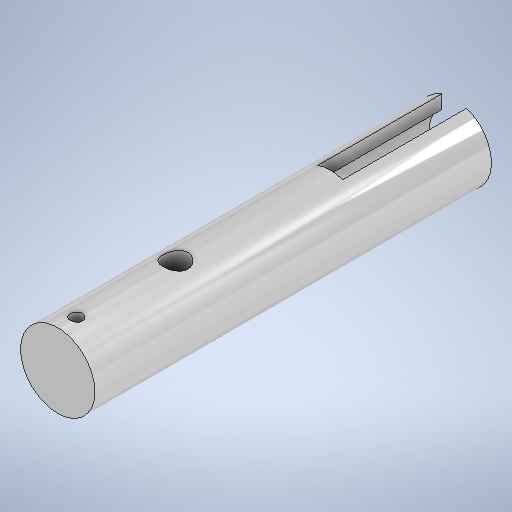
# Autodesk Inventor part: small_bar_motor
Saved by Autodesk Inventor 2025.1 (Build 291241000, 241)
## iProperties
Created: 2022-02-09
Part Number: small_bar_motor
Material: アルミニウム 6061-AHC
Document SubType Name: Modeling
Designer: 中島 青蔵
Density: 2.7 g/cm^3
Appearance: アルミニウム - ダーク
Author: 中島 青蔵
Autodesk Inventor part; units mm, degrees
ref_plane "YZ Plane" through (0, 0, 0) normal (1, 0, 0) x (0, 1, 0)
ref_plane "XY Plane" through (0, 0, 0) normal (0, 0, 1) x (1, 0, 0)
sketch "スケッチ1" plane through (0, 0, 0) normal (0, 0, 1) x (1, 0, 0)
  circle A0 centre (0, 0) radius 6
  dimension "d0" = 12
  constraints: 1 centre point, 1 coincident
  measures "d0" diameter of A0
extrude "押し出し1" add sketch "スケッチ1" along normal blind 64
ref_plane "作業平面1" through (0, 6, 0) normal (0, 1, 0) x (-1, 0, 0)
sketch "スケッチ2" plane through (0, 6, 0) normal (0, 1, 0) x (-1, 0, 0)
  line L0 (0, 0) -> (2, 0)
  line L1 (2, 0) -> (2, 20)
  line L2 (2, 20) -> (0, 20)
  line L3 (0, 20) -> (0, 0)
  line L4 (6, 0) -> (-6, 0) projected
  line L5 (0, 20) -> (-2, 20)
  line L6 (-2, 20) -> (-2, 0)
  line L7 (-2, 0) -> (0, 0)
  line L8 (0, 0) -> (0, 20)
  dimension "d3" = 2
  dimension "d4" = 20
  dimension "d5" = 2
  dimension "d31" = 4
  constraints: 16 end point, 1 point on line
  measures "d3" distance of L2.end L1.end
  measures "d4" distance of L1.end L0.end
  measures "d5" distance of L7.end L6.end
  measures "d31" distance between parallel lines of L1 L6
extrude "押し出し2" cut sketch "スケッチ2" against normal blind 6
sketch "スケッチ3" plane through (0, 0, 0) normal (0, 0, -1) x (-1, 0, 0)
  point P0 (0, 0)
  point P1 (0, 0)
  constraints: 1 coincident
hole "穴1" at (0, 0, 0) direction (0, 0, 1) diameter 8 depth 20 tip angle 118
sketch "スケッチ4" plane through (0, 6, 0) normal (0, 1, 0) x (-1, 0, 0)
  line L0 (2, 20) -> (-2, 20) projected
  point P0 (0, 0)
  point P1 (0, 45)
  dimension "d15" = 25
  measures "d15" distance from line of point (0, 45) L0
hole "穴2" at (0, 6, 45) direction (0, -1, 0) diameter 4 end through all
sketch "スケッチ5" plane through (0, 6, 0) normal (0, 1, 0) x (-1, 0, 0)
  line L0 (6, 64) -> (-6, 64) projected
  point P0 (0, 0)
  point P1 (0, 61)
  dimension "d23" = 3
  measures "d23" distance from line of L0 point (0, 61)
hole "穴3" at (0, 6, 61) direction (0, -1, 0) diameter 2 end through all
